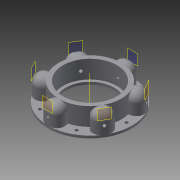
# Autodesk Inventor part: flangev6
Saved by Autodesk Inventor 2015 (Build 190159000, 159)
## iProperties
Created: 2016-04-16
Part Number: flangev6
Material: Generic
Document SubType Name: Modeling
Designer: ypatel4
Density: 1 g/cm^3
Appearance: Default
Author: ypatel4
Autodesk Inventor part; units mm, degrees
ref_plane "YZ Plane" through (0, 0, 0) normal (1, 0, 0) x (0, 1, 0)
ref_plane "XZ Plane" through (0, 0, 0) normal (0, 1, 0) x (-1, 0, 0)
ref_plane "XY Plane" through (0, 0, 0) normal (0, 0, 1) x (1, 0, 0)
sketch "Sketch1" plane through (0, 0, 0) normal (0, 1, 0) x (-1, 0, 0)
  circle A0 centre (0, 0) radius 51.1302
  circle A1 centre (0, 0) radius 88.9
  dimension "d0" = 102.2604
  dimension "d1" = 177.8
  constraints: 2 centre point, 2 coincident
  measures "d0" diameter of A0
  measures "d1" diameter of A1
extrude "Extrusion1" add sketch "Sketch1" along normal blind 5.08
sketch "Sketch2" plane through (0, 5.08, 0) normal (0, 1, 0) x (1, 0, 0)
  circle A0 centre (0, 0) radius 66.167
  circle A1 centre (0, 0) radius 57.15
  dimension "d4" = 132.334
  dimension "d47" = 114.3
  constraints: 2 centre point, 2 coincident
  measures "d4" diameter of A0
  measures "d47" diameter of A1
extrude "Extrusion4" add sketch "Sketch2" along normal blind 38.1
sketch "Sketch9" plane through (0, 5.08, 0) normal (0, 1, 0) x (1, 0, 0)
  circle A0 centre (0, 0) radius 88.9 construction
  circle A1 centre (0, 0) radius 66.167 construction
  line L0 (66.167, 0) -> (88.9, 0) construction
  line L1 (77.5335, -8.0816) -> (77.5335, 0) construction
  line L2 (77.5335, 0) -> (77.5335, 5.6242) construction
  circle A2 centre (77.5335, 0) radius 3.175
  dimension "d52" = 22.733
  dimension "d54" = 6.35
  constraints: 6 end point, 2 horizontal alignment, 2 perpendicular, 2 vertical, 1 centre point, 1 coincident, 1 horizontal, 1 midpoint, 2 other
  measures "d52" distance of L0.start L0.end
  measures "d54" diameter of A2
hole "Hole4" at (77.5335, 5.08, 0) direction (0, -1, 0) diameter 6.35 end through all
pattern_circular "Circular Pattern4" count 6 over 360 about axis through (0, -10, 0) along (0, 1, 0) of "Hole4"
sketch "Sketch11" plane through (0, 5.08, 0) normal (0, 1, 0) x (1, 0, 0)
  circle A0 centre (0, 0) radius 88.9 projected
  circle A1 centre (0, 0) radius 66.167 projected
  circle A2 centre (0, 0) radius 88.9 projected
  circle A3 centre (0, 0) radius 66.167 projected
  line L0 (46.6635, 46.9105) -> (63.8491, 61.8587)
  line L1 (63.9331, 17.0478) -> (86.2859, 21.3997)
  dimension "d71" = 30
  constraints: 8 point on circle, 4 end point
  measures "d71" angle of L1 L0
extrude "Extrusion5" add sketch "Sketch11" along normal blind 38.1 contours L1 A1 L0 A0 picked at (77.6501, 23.662)
ref_plane "Work Plane4" through (77.7455, 43.18, -43.1143) normal (0.8745279, 0, -0.4849752) x (0, 1, 0)
sketch "Sketch12" plane through (77.7455, 43.18, -43.1143) normal (0.8745279, 0, -0.4849752) x (0, 1, 0)
  line L0 (0, 57.15) -> (0, -57.15) projected
  line L1 (0, 0) -> (-21.59, 0) construction
  circle A0 centre (-21.59, 0) radius 3.175
  point P0 (-43.18, 0)
  dimension "d74" = 21.59
  dimension "d75" = 6.35
  constraints: 2 end point, 1 centre point, 1 coincident, 1 horizontal, 1 midpoint
  measures "d74" distance of L1.start L1.end
  measures "d75" diameter of A0
hole "Hole5" at (77.7455, 21.59, -43.1143) direction (-0.8745279, 0, 0.4849752) diameter 6.35 depth 50.8
fillet "Fillet1" radius 15.875 5 edges at (55.2563, 43.18, -54.3846) (63.8491, 24.13, -61.8587) (77.7455, 43.18, -43.1143) (75.1095, 43.18, -19.2237) (86.2859, 24.13, -21.3997)
pattern_circular "Circular Pattern6" count 6 over 360 about axis through (0, -10, 0) along (0, 1, 0) of "Extrusion5", "Hole5", "Fillet1"
sketch "Sketch3" plane through (0, 5.08, 0) normal (0, 1, 0) x (1, 0, 0)
  circle A0 centre (0, 0) radius 66.167 projected
  circle A1 centre (0, 0) radius 88.9 projected
  circle A2 centre (0, 0) radius 66.167 projected
  line L0 (66.167, 0) -> (88.9, 0) construction
  circle A3 centre (77.5335, 0) radius 3.175
  dimension "d50" = 22.733
  dimension "d51" = 6.35
  constraints: 3 horizontal alignment, 2 end point, 1 centre point, 1 coincident, 1 horizontal, 3 other
  measures "d50" distance of L0.start L0.end
  measures "d51" diameter of A3
sketch "Sketch4" plane through (0, 5.08, 0) normal (0, 1, 0) x (1, 0, 0)
  line L0 (43.7224, 49.663) -> (63.9658, 61.7381)
  circle A0 centre (0, 0) radius 88.9 projected
  line L1 (64.5027, 14.7461) -> (84.7557, 26.8269)
  arc A1 (81.2449, 36.0899) -> (63.9658, 61.7381) centre (0, 0) ccw
  circle A2 centre (77.5335, 0) radius 3.175 projected
  circle A3 centre (38.7668, 67.146) radius 3.175 projected
  circle A4 centre (0, 0) radius 66.167 projected
  constraints: 5 point on circle, 4 end point, 1 centre point, 1 concentric, 1 parallel
sketch "Sketch6" plane through (-63.9658, 43.434, 61.7381) normal (-0.719525, 0, 0.6944666) x (0, -1, 0)
  line L0 (0, 51.1302) -> (0, -51.1302) projected
  line L1 (0, 0) -> (-21.717, 0)
  circle A0 centre (-21.717, 0) radius 3.175
  point P0 (43.434, 0)
  dimension "d35" = 21.717
  dimension "d36" = 6.35
  constraints: 2 end point, 1 centre point, 1 coincident, 1 horizontal, 1 midpoint
  measures "d35" distance of L1.start L1.end
  measures "d36" diameter of A0
ref_plane "Work Plane5" through (1.5347, 43.18, -88.8868) normal (0.0172632, 0, -0.999851) x (0, 1, 0)
ref_plane "Work Plane6" through (-76.2108, 43.18, -45.7725) normal (-0.8572648, 0, -0.5148758) x (0, 1, 0)
ref_plane "Work Plane7" through (-77.7455, 43.18, 43.1143) normal (-0.8745279, 0, 0.4849752) x (0, 1, 0)
ref_plane "Work Plane8" through (-1.5347, 43.18, 88.8868) normal (-0.0172632, 0, 0.999851) x (0, 1, 0)
ref_plane "Work Plane9" through (76.2108, 43.18, 45.7725) normal (0.8572648, 0, 0.5148758) x (0, 1, 0)
body "Solid1"
